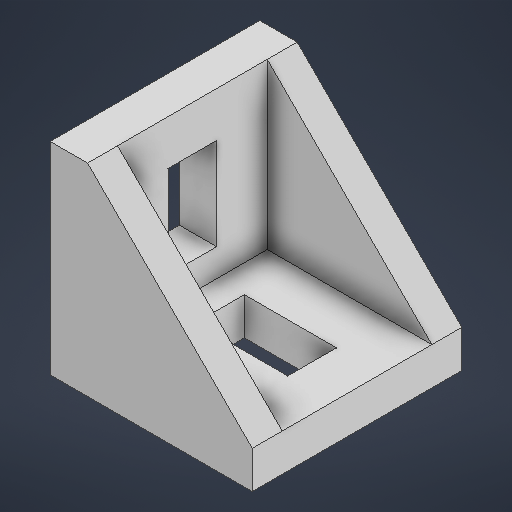
# Autodesk Inventor part: masterpiece_uhelnik
Saved by Autodesk Inventor 2025.1 (Build 291241000, 241)
## iProperties
Created: 2024-12-16
Part Number: masterpiece_uhelnik
Material: Všeobecné
Document SubType Name: Modeling
Designer: lukas
Density: 1 g/cm^3
Appearance: Výchozí
Author: lukas
## iProperties of the stored document masterpiece_uhelnik_3D tisk.ipt
Created: 2024-12-16
Part Number: masterpiece_uhelnik_3D tisk
Material: Všeobecné
Document SubType Name: Modeling
Designer: lukas
Density: 1 g/cm^3
Appearance: Výchozí
Author: lukas
Autodesk Inventor part; units mm, degrees
ref_plane "YZ Plane" through (0, 0, 0) normal (1, 0, 0) x (0, 1, 0)
ref_plane "XZ Plane" through (0, 0, 0) normal (0, 1, 0) x (-1, 0, 0)
ref_plane "XY Plane" through (0, 0, 0) normal (0, 0, 1) x (1, 0, 0)
sketch "Náčrt1" plane through (0, 0, 0) normal (0, 0, 1) x (1, 0, 0)
  line L0 (-18.9, 0) -> (18.9, 0) projected
  line L1 (0, 18.9) -> (0, -18.9) projected
  line L2 (-13.5, -13.5) -> (13.5, -13.5)
  line L3 (13.5, -13.5) -> (13.5, -8.5)
  line L4 (13.5, -8.5) -> (-8.5, 13.5)
  line L5 (-8.5, 13.5) -> (-13.5, 13.5)
  line L6 (-13.5, 13.5) -> (-13.5, -13.5)
  point P0 (0, 0)
  dimension "d0" = 27
  dimension "d1" = 27
  dimension "d2" = 5
  dimension "d3" = 5
  constraints: 10 end point, 2 perpendicular, 1 horizontal, 1 vertical, 2 other
  measures "d0" distance of L5.end L2.start
  measures "d1" distance of L2.start L2.end
  measures "d2" distance of L2.end L3.end
  measures "d3" distance of L4.end L5.end
extrude "Vysunutí1" add sketch "Náčrt1" along normal blind 28
ref_plane "Pracovní rovina3" through (13.5, -13.5, 0) normal (-1, 0, 0) x (0, 0, 1)
sketch "Náčrt5" plane through (13.5, -13.5, 0) normal (-1, 0, 0) x (0, 0, 1)
  line L0 (0, 5) -> (0, 27) projected
  line L1 (0, 27) -> (28, 27) projected
  line L2 (28, 5) -> (28, 27) projected
  line L3 (0, 5) -> (28, 5) projected
  line L4 (24, 27) -> (4, 27)
  line L5 (4, 27) -> (4, 5)
  line L6 (4, 5) -> (24, 5)
  line L7 (24, 5) -> (24, 27)
  point P0 (0, 13.5)
  dimension "d24" = 20
  dimension "d25" = 4
  constraints: 8 end point, 2 parallel, 2 point on line, 1 horizontal, 1 perpendicular
  measures "d24" distance between parallel lines of L7 L5
  measures "d25" distance between parallel lines of L0 L5
extrude "Vysunutí5" cut sketch "Náčrt5" along normal blind 22 contours L5 L1 L7 L3
sketch "Náčrt6" plane through (-13.5, -13.5, 0) normal (-1, 0, 0) x (0, 0, 1)
  line L0 (0, 27) -> (0, 0) projected
  line L1 (0, 0) -> (28, 0) projected
  line L2 (28, 27) -> (28, 0) projected
  line L3 (0, 27) -> (28, 27) projected
  line L4 (10.75, 21) -> (17.25, 21)
  line L5 (17.25, 21) -> (17.25, 8.7)
  line L6 (17.25, 8.7) -> (10.75, 8.7)
  line L7 (10.75, 8.7) -> (10.75, 21)
  point P0 (0, 13.5)
  dimension "d28" = 6.5
  dimension "d29" = 12.3
  dimension "d30" = 10.75
  dimension "d31" = 6
  constraints: 8 end point, 2 parallel, 1 horizontal, 1 perpendicular
  measures "d28" distance of L4.start L4.end
  measures "d29" distance of L4.end L5.end
  measures "d30" distance between parallel lines of L0 L7
  measures "d31" distance between parallel lines of L3 L4
extrude "Vysunutí6" cut sketch "Náčrt6" against normal through all contours L4 L5 L6 L7
pattern_circular "Kruhové pole1" count 2 over 90 about axis through (-13.5, -13.5, 0) along (0, 0, -1) of "Vysunutí6"
sketch "Náčrt7" plane through (-13.5, -13.5, 0) normal (0, -1, 0) x (1, 0, 0)
  line L0 (0, 0) -> (27, 0) projected
  line L1 (27, 0) -> (27, 28) projected
  line L2 (0, 28) -> (27, 28) projected
  line L3 (0, 0) -> (0, 28) projected
  line L4 (-5.4, 0) -> (32.4, 0) projected
  line L5 (-5.4, 0) -> (32.4, 0) projected
  line L6 (13.5, -5.6) -> (13.5, 33.6) projected
  line L7 (21, 17.25) -> (8.7, 17.25)
  line L8 (8.7, 17.25) -> (8.7, 10.75)
  line L9 (8.7, 10.75) -> (21, 10.75)
  line L10 (21, 10.75) -> (21, 17.25)
  point P0 (13.5, 0)
  dimension "d37" = 12.3
  dimension "d38" = 6.5
  dimension "d39" = 6
  dimension "d40" = 10.75
  constraints: 8 end point, 2 parallel, 1 horizontal, 1 perpendicular
  measures "d37" distance of L9.end L8.end
  measures "d38" distance of L8.end L7.end
  measures "d39" distance between parallel lines of L1 L10
  measures "d40" distance between parallel lines of L2 L7
extrude "Vysunutí7" cut sketch "Náčrt7" against normal through all contours L9 L8 L7 L6 | L6 L7 L10 L9
